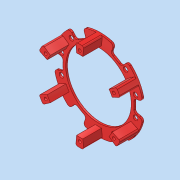
# Autodesk Inventor part: retentionStandoff
Saved by Autodesk Inventor 2017 (Build 210142000, 142)
## iProperties
Created: 2016-11-29
Part Number: retentionStandoff
Material: ABS Plastic
Document SubType Name: Modeling
Designer: techn
Density: 1.06 g/cm^3
Appearance: Light Red
Mass: 12.5265 g
Surface Area: 109.755 cm^2
Volume: 11.8175 cm^3
Author: techn
Autodesk Inventor part; units mm, degrees
ref_plane "YZ Plane" through (0, 0, 0) normal (1, 0, 0) x (0, 1, 0)
ref_plane "XZ Plane" through (0, 0, 0) normal (0, 1, 0) x (-1, 0, 0)
ref_plane "XY Plane" through (0, 0, 0) normal (0, 0, 1) x (1, 0, 0)
sketch "Sketch2" plane through (0, 0, 0) normal (0, 0, 1) x (1, 0, 0)
  circle A0 centre (0, 0) radius 34.925
  circle A1 centre (0, 0) radius 47.625
  dimension "d12" = 69.85
  dimension "d13" = 95.25
  constraints: 2 centre point, 2 coincident
  measures "d12" diameter of A0
  measures "d13" diameter of A1
extrude "Extrusion2" add sketch "Sketch2" along normal blind 1.905
sketch "Sketch3" plane through (0, 0, 1.905) normal (0, 0, 1) x (1, 0, 0)
  line L0 (0, 0) -> (0, 41.91)
  circle A0 centre (0, 41.91) radius 1.5875
  line L1 (0, 0) -> (3.0439, 34.7921)
  circle A1 centre (0, 0) radius 34.925 projected
  line L2 (0, 0) -> (34.925, 0) construction
  line L3 (0, 0) -> (-3.0439, 34.7921)
  line L4 (0, 0) -> (34.925, 0) construction
  line L5 (-3.0439, 34.7921) -> (-4.1508, 47.4438)
  circle A2 centre (0, 0) radius 47.625 projected
  line L6 (3.0439, 34.7921) -> (4.1508, 47.4438)
  dimension "d16" = 41.91
  dimension "d17" = 3.175
  dimension "d18" = 85
  dimension "d19" = 95
  constraints: 14 end point, 4 point on circle, 2 equal length, 2 horizontal, 1 centre point, 1 coincident, 1 collinear, 1 point on line, 1 vertical
  measures "d16" distance of L0.start L0.end
  measures "d17" diameter of A0
  measures "d18" angle of L2 L1
  measures "d19" angle of L4 L3
extrude "Extrusion3" add sketch "Sketch3" along normal blind 19.9644 contours A1 L5 A2 L6 picked at (2.9141, 41.2642)
pattern_circular "Circular Pattern1" count 6 over 360 about axis through (0, 0, 0) along (0, 0, 1) of "Extrusion3"
sketch "Sketch4" plane through (0, 0, 1.905) normal (0, 0, 1) x (1, 0, 0)
  line L0 (0, 0) -> (30.6128, 36.4829)
  arc A0 (39.0121, 27.3166) -> (4.1508, 47.4438) centre (0, 0) ccw projected
  line L1 (0, 0) -> (47.625, 0) construction
  line L2 (0, 0) -> (16.2887, 44.7529)
  line L3 (0, 0) -> (47.625, 0) construction
  arc A1 (24.4902, 29.1863) -> (13.031, 35.8023) centre (-19.1955, -33.2476) ccw
  dimension "d25" = 50
  dimension "d26" = 70
  dimension "d27" = 76.2
  dimension "d28" = 38.1
  dimension "d35" = 38.1
  constraints: 8 end point, 4 point on circle, 2 equal length, 2 horizontal, 2 point on line, 1 centre point
  measures "d25" angle of L1 L0
  measures "d26" angle of L3 L2
  measures "d27" radius of A1
  measures "d28" distance of L0.start A1.end
  measures "d35" distance of L0.start A1.start
extrude "Extrusion4" cut sketch "Sketch4" against normal blind 25.4 contours A1 L2 A0 L0
pattern_circular "Circular Pattern2" count 6 over 360 about axis through (0, 0, 0) along (0, 0, 1) of "Extrusion4"
sketch "Sketch5" plane through (0, 0, 1.905) normal (0, 0, 1) x (1, 0, 0)
  circle A0 centre (0, 0) radius 38.1
  dimension "d34" = 76.2
  constraints: 1 centre point, 1 coincident
  measures "d34" diameter of A0
extrude "Extrusion5" cut sketch "Sketch5" along normal blind 25.4
sketch "Sketch6" plane through (0, 0, 1.905) normal (0, 0, 1) x (1, 0, 0)
  line L0 (0, 0) -> (39.3779, 10.5513)
  line L1 (0, 0) -> (40.767, 0) construction
  circle A0 centre (39.3779, 10.5513) radius 2.54
  line L2 (0, 0) -> (0, 16.1811)
  circle A1 centre (39.3779, -10.5513) radius 2.54
  circle A2 centre (-39.3779, 10.5513) radius 2.54
  circle A3 centre (-39.3779, -10.5513) radius 2.54
  line L3 (0, 0) -> (28.8266, 28.8266)
  line L4 (0, 0) -> (40.767, 0) construction
  circle A4 centre (28.8266, 28.8266) radius 2.54
  circle A5 centre (-28.8266, 28.8266) radius 2.54
  dimension "d38" = 40.767
  dimension "d39" = 15
  dimension "d40" = 5.08
  dimension "d43" = 40.767
  dimension "d44" = 45
  dimension "d45" = 5.08
  constraints: 10 end point, 6 centre point, 4 symmetric about line, 2 coincident, 2 equal length, 2 horizontal, 1 vertical, 4 other
  measures "d38" distance of L0.start L0.end
  measures "d39" angle of L1 L0
  measures "d40" diameter of A0
  measures "d43" distance of L0.start L3.end
  measures "d44" angle of L4 L3
  measures "d45" diameter of A4
extrude "Extrusion6" cut sketch "Sketch6" against normal blind 25.4 contours A0 | A1 | A2 | A3
extrude "Extrusion7" cut sketch "Sketch6" against normal blind 25.4 contours A4 | A5
fillet "Fillet1" radius 1.5875 12 edges at (39.0121, 27.3166, 11.8872) (43.1629, 20.1272, 11.8872) (4.1508, 47.4438, 11.8872) (-4.1508, 47.4438, 11.8872) (-39.0121, 27.3166, 11.8872) (-43.1629, 20.1272, 11.8872) (-43.1629, -20.1272, 11.8872) (-39.0121, -27.3166, 11.8872) (-4.1508, -47.4438, 11.8872) (4.1508, -47.4438, 11.8872) (43.1629, -20.1272, 11.8872) (39.0121, -27.3166, 11.8872)
fillet "Fillet2" radius 3.175 24 edges at (30.6128, 36.4829, 0.9525) (24.4902, 29.1863, 0.9525) (16.2887, 44.7529, 0.9525) (13.031, 35.8023, 0.9525) (-16.2887, 44.7529, 0.9525) (-24.4902, 29.1863, 0.9525) (-30.6128, 36.4829, 0.9525) (-13.031, 35.8023, 0.9525) (-46.9015, 8.27, 0.9525) (-37.5212, 6.616, 0.9525) (-37.5212, -6.616, 0.9525) (-46.9015, -8.27, 0.9525) (-16.2887, -44.7529, 0.9525) (-13.031, -35.8023, 0.9525) (-24.4902, -29.1863, 0.9525) (-30.6128, -36.4829, 0.9525) (30.6128, -36.4829, 0.9525) (16.2887, -44.7529, 0.9525) (24.4902, -29.1863, 0.9525) (13.031, -35.8023, 0.9525) (46.9015, -8.27, 0.9525) (46.9015, 8.27, 0.9525) (37.5212, 6.616, 0.9525) (37.5212, -6.616, 0.9525)
body "Solid2"
